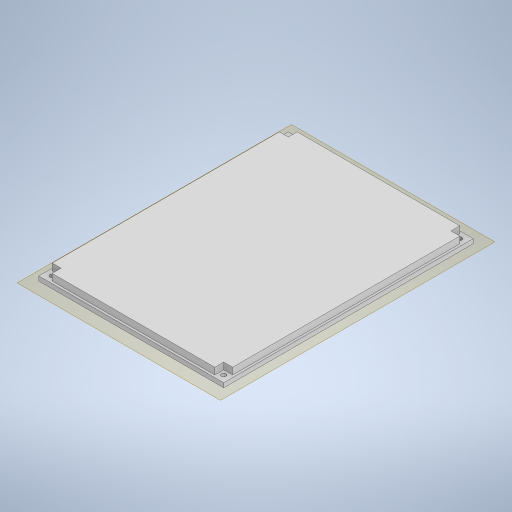
# Autodesk Inventor part: bottom plant watner
Saved by Autodesk Inventor 2024 (Build 280153000, 153)
## iProperties
Created: 2024-03-17
Part Number: bottom plant watner
Material: Generic
Document SubType Name: Modeling
Designer: Emil
Density: 1 g/cm^3
Appearance: Default
Author: Emil
Autodesk Inventor part; units mm, degrees
ref_plane "YZ Plane" through (0, 0, 0) normal (1, 0, 0) x (0, 1, 0)
ref_plane "XY Plane" through (0, 0, 0) normal (0, 0, 1) x (1, 0, 0)
sketch "Sketch7" plane through (0, 0, 0) normal (0, 1, 0) x (-1, 0, 0)
  line L0 (-41.5, 56) -> (41.5, 56)
  line L1 (41.5, 56) -> (41.5, -56)
  line L2 (41.5, -56) -> (-41.5, -56)
  line L3 (-41.5, -56) -> (-41.5, 56)
  line L4 (-41.5, 56) -> (41.5, -56) construction
  line L5 (41.5, 56) -> (-41.5, -56) construction
  line L6 (-40.5, 55) -> (40.5, -55) construction
  line L7 (40.5, 55) -> (-40.5, -55) construction
  line L8 (36.5, 55) -> (36.5, 51)
  line L9 (36.5, 51) -> (40.5, 51)
  line L10 (36.5, -55) -> (36.5, -51)
  line L11 (36.5, -51) -> (40.5, -51)
  line L12 (-36.5, -55) -> (-36.5, -51)
  line L13 (-36.5, -51) -> (-40.5, -51)
  line L14 (-36.5, 55) -> (-36.5, 51)
  line L15 (-36.5, 51) -> (-40.5, 51)
  line L16 (40.5, -51) -> (40.5, 51)
  line L17 (36.5, 55) -> (-36.5, 55)
  line L18 (-40.5, 51) -> (-40.5, -51)
  line L19 (-36.5, -55) -> (36.5, -55)
  circle A0 centre (38.5, 53) radius 1
  circle A1 centre (38.5, -53) radius 1
  circle A2 centre (-38.5, 53) radius 1
  circle A3 centre (-38.5, -53) radius 1
  point P0 (0, 0)
  dimension "d36" = 83
  dimension "d37" = 112
  dimension "d38" = 81
  dimension "d39" = 110
  dimension "d40" = 4
  dimension "d41" = 4
  dimension "d42" = 4
  dimension "d43" = 4
  dimension "d44" = 4
  dimension "d45" = 4
  dimension "d46" = 4
  dimension "d47" = 4
  dimension "d48" = 2
  dimension "d49" = 2
  dimension "d50" = 2
  dimension "d51" = 2
  constraints: 40 end point, 4 centre point, 4 midpoint, 4 parallel, 3 perpendicular, 1 horizontal
  measures "d36" distance of L1.end L2.end
  measures "d37" distance of L0.end L1.end
  measures "d38" distance of L6.end L7.end
  measures "d39" distance of L7.start L6.end
  measures "d40" distance of L9.end L8.end
  measures "d41" distance of L8.end L8.start
  measures "d42" distance of L10.end L11.end
  measures "d43" distance of L10.start L10.end
  measures "d44" distance of L13.end L12.end
  measures "d45" distance of L12.end L12.start
  measures "d46" distance of L14.end L15.end
  measures "d47" distance of L14.start L14.end
  measures "d48" diameter of A0
  measures "d49" diameter of A1
  measures "d50" diameter of A2
  measures "d51" diameter of A3
extrude "Extrusion4" add sketch "Sketch7" along normal blind 2
sketch "Sketch8" plane through (0, 0, 0) normal (0, 1, 0) x (-1, 0, 0)
  point P0 (0, 0)
sketch "Sketch9" plane through (0, 0, 0) normal (0, 1, 0) x (-1, 0, 0)
  line L0 (36.5, 55) -> (36.5, 51) projected
  line L1 (36.5, 51) -> (40.5, 51) projected
  line L2 (36.5, 51) -> (40.5, 51)
  line L3 (40.5, -51) -> (36.5, -51) projected
  line L4 (40.5, 51) -> (40.5, -51)
  line L5 (40.5, -51) -> (36.5, -51)
  line L6 (36.5, -51) -> (36.5, -55) projected
  line L7 (36.5, -51) -> (36.5, -55)
  line L8 (36.5, -55) -> (-36.5, -55) projected
  line L9 (36.5, -55) -> (-36.5, -55)
  line L10 (-36.5, -55) -> (-36.5, -51)
  line L11 (-40.5, -51) -> (-40.5, 51) projected
  line L12 (-36.5, -51) -> (-40.5, -51)
  line L13 (-40.5, -51) -> (-40.5, 51)
  line L14 (-40.5, 51) -> (-36.5, 51) projected
  line L15 (-40.5, 51) -> (-36.5, 51)
  line L16 (-36.5, 55) -> (36.5, 55) projected
  line L17 (-36.5, 51) -> (-36.5, 55)
  line L18 (-36.5, 55) -> (36.5, 55)
  line L19 (36.5, 55) -> (36.5, 51)
  point P0 (0, 0)
  constraints: 24 end point, 9 perpendicular, 3 collinear, 1 point on line
extrude "Extrusion5" add sketch "Sketch9" along normal blind 5
body "Solid2"
